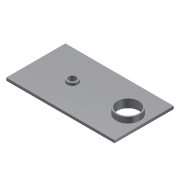
# Autodesk Inventor part: Cover
Saved by Autodesk Inventor 2012 (Build 160160000, 160)
## iProperties
Created: 2017-01-27
Part Number: Cover
Material: Default
Document SubType Name: Modeling
Designer: omaro
Density: 1 g/cm^3
Author: omaro
Autodesk Inventor part; units mm, degrees
ref_plane "YZ Plane" through (0, 0, 0) normal (1, 0, 0) x (0, 1, 0)
ref_plane "XZ Plane" through (0, 0, 0) normal (0, 1, 0) x (-1, 0, 0)
ref_plane "XY Plane" through (0, 0, 0) normal (0, 0, 1) x (1, 0, 0)
sketch "Sketch1" plane through (0, 0, 0) normal (0, 0, 1) x (1, 0, 0)
  line L0 (-14.5985, 9.3978) -> (106.6015, 9.3978)
  line L1 (106.6015, 9.3978) -> (106.6015, -56.8022)
  line L2 (106.6015, -56.8022) -> (-14.5985, -56.8022)
  line L3 (-14.5985, -56.8022) -> (-14.5985, 9.3978)
  circle A0 centre (88.6015, -23.7022) radius 11.9
  circle A1 centre (26.4015, -23.7022) radius 4
  point P0 (0, 0)
  dimension "d0" = 121.2
  dimension "d1" = 66.2
  dimension "d3" = 33.1
  dimension "d4" = 8
  dimension "d5" = 23.8
  dimension "d6" = 18
  dimension "d7" = 41
  constraints: 8 end point, 2 centre point, 2 parallel, 1 horizontal, 1 perpendicular
  measures "d0" distance of L0.start L0.end
  measures "d1" distance of L2.end L0.start
  measures "d3" distance from line of L0 A1.centre
  measures "d4" diameter of A1
  measures "d5" diameter of A0
  measures "d6" distance from line of L1 A0.centre
  measures "d7" distance from line of L3 A1.centre
extrude "Extrusion1" add sketch "Sketch1" along normal mid plane 3
sketch "Sketch2" plane through (0, 0, 1.5) normal (0, 0, 1) x (1, 0, 0)
  circle A0 centre (26.4015, -23.7022) radius 4 projected
  circle A1 centre (26.4015, -23.7022) radius 6
  point P0 (0, 0)
  dimension "d10" = 12
  constraints: 1 centre point, 1 coincident
  measures "d10" diameter of A1
extrude "Extrusion2" add sketch "Sketch2" along normal blind 3
sketch "Sketch3" plane through (0, 0, 1.5) normal (0, 0, 1) x (1, 0, 0)
  circle A0 centre (88.6015, -23.7022) radius 11.9 projected
  circle A1 centre (88.6015, -23.7022) radius 13.4
  point P0 (0, 0)
  dimension "d13" = 23.8
  dimension "d14" = 26.8
  constraints: 1 centre point, 1 coincident
  measures "d13" diameter of A0
  measures "d14" diameter of A1
extrude "Extrusion3" add sketch "Sketch3" along normal blind 6.4
equation "\"d3\" = 0.5 * d1"
body "Solid1"
